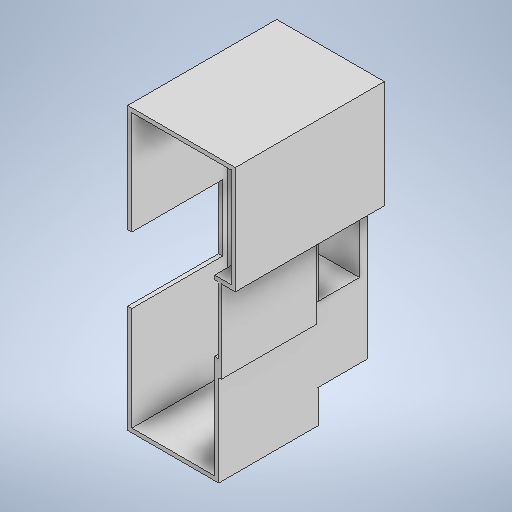
# Autodesk Inventor part: InjectionMachine
Saved by Autodesk Inventor 2025.1 (Build 291241000, 241)
## iProperties
Created: 2025-01-30
Part Number: InjectionMachine
Material: Generic
Document SubType Name: Modeling
Designer: yovan
Density: 1 g/cm^3
Appearance: Default
Author: yovan
Autodesk Inventor part; units mm, degrees
ref_plane "YZ Plane" through (0, 0, 0) normal (1, 0, 0) x (0, 1, 0)
ref_plane "XZ Plane" through (0, 0, 0) normal (0, 1, 0) x (-1, 0, 0)
ref_plane "XY Plane" through (0, 0, 0) normal (0, 0, 1) x (1, 0, 0)
sketch "Sketch1" plane through (0, 0, 0) normal (0, 0, 1) x (1, 0, 0)
  line L0 (0, 0) -> (1300, 0)
  line L1 (1300, 3400) -> (0, 3400)
  line L2 (0, 3400) -> (0, 0)
  line L3 (1300, 2100) -> (1100, 2100)
  line L4 (1100, 2100) -> (1100, 0)
  line L5 (1300, 2100) -> (1300, 3400)
  dimension "d0" = 1300
  constraints: 12 end point, 3 perpendicular, 2 parallel, 1 horizontal, 1 point on line
  measures "d0" distance of L1.end L1.start
extrude "Extrusion1" add sketch "Sketch1" along normal blind 1800
sketch "Sketch2" plane through (0, 0, 0) normal (-1, 0, 0) x (0, 0, 1)
  line L0 (0, 0) -> (1800, 0) projected
  line L1 (0, 0) -> (600, 0)
  line L2 (600, 0) -> (600, 400)
  line L3 (600, 400) -> (0, 400)
  line L4 (0, 400) -> (0, 0)
  line L5 (0, 3400) -> (1800, 3400) projected
  line L6 (0, 1300) -> (600, 1300)
  line L7 (600, 1300) -> (600, 2100)
  line L8 (600, 2100) -> (0, 2100)
  line L9 (0, 2100) -> (0, 1300)
  line L10 (600, 1300) -> (100, 1300)
  line L11 (100, 1300) -> (100, 2100)
  line L12 (100, 2100) -> (600, 2100)
  line L13 (600, 2100) -> (600, 1300)
  line L14 (600, 1300) -> (600, 400)
  line L15 (700, 2100) -> (1800, 2100)
  line L16 (1800, 2100) -> (1800, 1300)
  line L17 (1800, 1300) -> (700, 1300)
  line L18 (700, 1300) -> (700, 2100)
  dimension "d4" = 600
  dimension "d5" = 400
  dimension "d13" = 600
  dimension "d14" = 800
  dimension "d15" = 500
  dimension "d21" = 900
  dimension "d25" = 800
  constraints: 34 end point, 8 parallel, 4 horizontal, 4 perpendicular, 1 point on line
  measures "d4" distance of L3.end L2.end
  measures "d5" distance of L2.end L1.end
  measures "d13" distance of L8.end L7.end
  measures "d14" distance of L7.end L6.end
  measures "d15" distance of L11.end L12.end
  measures "d21" distance of L6.end L2.end
  measures "d25" distance of L15.end L16.end
extrude "Extrusion2" cut sketch "Sketch2" against normal blind 1800 contours L4 L3 L2 L0 | L11 L8 L7 L6 | L15 L16 L17 L18
sketch "Sketch3" plane through (0, 0, 1800) normal (0, 0, 1) x (1, 0, 0)
  line L0 (50, 2400) -> (50, 49.9974)
  line L1 (50, 49.9974) -> (1050, 49.9974)
  line L2 (1050, 49.9974) -> (1050, 2150)
  line L3 (1050, 2100) -> (1050, 2150)
  line L4 (1100, 2100) -> (1300, 2100) projected
  line L5 (0, 3400) -> (0, 2100) projected
  line L6 (0, 2100) -> (0, 3400)
  line L7 (0, 3400) -> (1300, 3400)
  line L8 (1300, 3400) -> (1300, 2100)
  line L9 (1250, 3350) -> (50, 3350)
  line L10 (50, 3350) -> (50, 2150)
  line L11 (1050, 2150) -> (1250, 2150)
  line L12 (1250, 2150) -> (1250, 3350)
  line L13 (1300, 2100) -> (1250, 2100)
  dimension "d46" = 50
  constraints: 24 end point, 4 parallel, 2 perpendicular, 2 point on line, 1 horizontal, 1 other
  measures "d46" distance between parallel lines of L7 L9
extrude "Extrusion3" cut sketch "Sketch3" against normal blind 1150
sketch "Sketch6" plane through (0, 0, 650) normal (0, 0, 1) x (1, 0, 0)
  line L0 (1050, 1300) -> (1050, 49.9974) projected
  line L1 (0, 2100) -> (1100, 2100) projected
  line L2 (1050, 1300) -> (50, 1300)
  line L3 (50, 1300) -> (50, 2100)
  line L4 (50, 2100) -> (1050, 2100)
  line L5 (1050, 2100) -> (1050, 1300)
  line L6 (1050, 1700) -> (900, 1700)
  line L7 (900, 1700) -> (900, 2100)
  line L8 (900, 1700) -> (900, 1300)
  line L9 (50, 1700) -> (200, 1700)
  line L10 (200, 1700) -> (200, 1300)
  line L11 (200, 1700) -> (200, 2100)
  point P0 (0, 0)
  dimension "d32" = 1000
  dimension "d33" = 150
  dimension "d34" = 150
  constraints: 20 end point, 8 point on line, 3 perpendicular, 2 horizontal, 2 midpoint, 2 parallel
  measures "d32" distance of L3.end L4.end
  measures "d33" distance of L6.start L6.end
  measures "d34" distance of L9.start L9.end
extrude "Extrusion6" cut sketch "Sketch6" against normal blind 150 contours L1 L7 L8 L2 L10 L11
sketch "Sketch7" plane through (1100, 400, 0) normal (1, 0, 0) x (0, 0, -1)
  line L0 (-1800, 700) -> (-650, 700)
  line L1 (-650, -350.0026) -> (-650, 2950) projected
  line L2 (-650, 720) -> (-650, 700)
  line L3 (-650, 720) -> (-1800, 720)
  line L4 (-1800, 900) -> (-1800, -400) projected
  line L5 (-1800, 700) -> (-1800, 720)
  point P0 (0, -400)
  point P1 (-650, 2000)
  constraints: 8 end point, 3 point on line, 2 perpendicular, 1 collinear, 1 horizontal
extrude "Extrusion7" add sketch "Sketch7" along normal blind 30
sketch "Sketch8" plane through (1100, 1120, 1800) normal (0, 1, 0) x (1, 0, 0)
  line L0 (30, 0) -> (30, 1150) projected
  line L1 (0, 0) -> (0, 1150) projected
  line L2 (30, 1150) -> (0, 1150)
  line L3 (0, 1150) -> (0, 0)
  line L4 (0, 0) -> (30, 0)
  line L5 (30, 0) -> (30, 1150)
  point P0 (-1100, 1800)
  constraints: 8 end point, 2 parallel, 1 horizontal, 1 perpendicular
extrude "Extrusion8" add sketch "Sketch8" along normal blind 1000
sketch "Sketch9" plane through (1130, 400, 0) normal (1, 0, 0) x (0, 0, -1)
  line L0 (-650, 1700) -> (-650, 700) projected
  line L1 (-650, 1300) -> (-650, 1500)
  line L2 (-850, 1700) -> (-1050, 1700)
  arc A0 (-650, 1500) -> (-850, 1700) centre (-850, 1500) ccw
  line L3 (-650, 1700) -> (-1072.0308, 1700)
  line L4 (-1072.0308, 1700) -> (-1072.0308, 1153.2705)
  line L5 (-1072.0308, 1153.2705) -> (-650, 1153.2705)
  line L6 (-650, 1153.2705) -> (-650, 1700)
  point P0 (0, -400)
  dimension "d42" = 400
  dimension "d43" = 200
  constraints: 12 end point, 3 point on line, 2 parallel, 2 perpendicular, 2 point on circle, 2 tangent, 1 centre point, 1 collinear, 1 horizontal
  measures "d42" distance of L0.start L2.end
  measures "d43" radius of A0
extrude "Extrusion9" cut sketch "Sketch9" against normal blind 20 contours L0 A0 L3
body "Solid1"
